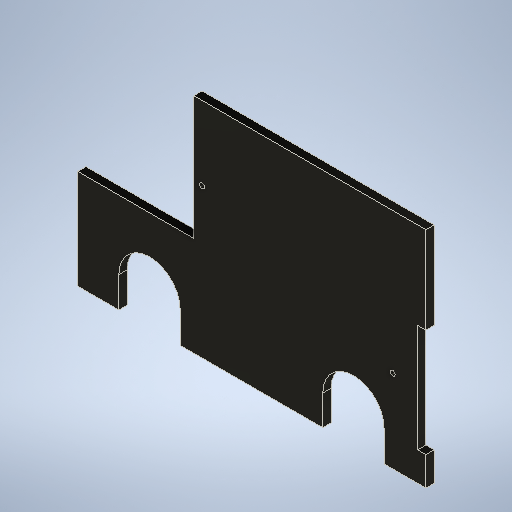
# Autodesk Inventor part: SIDE_1
Saved by Autodesk Inventor 2025.3 (Build 293356030, 356C)
## iProperties
Created: 2026-06-30
Part Number: SIDE_1
Material: ABS Plastic
Document SubType Name: Modeling
Designer: user
Density: 1.06 g/cm^3
Appearance: Gunmetal
Author: user
Autodesk Inventor part; units mm, degrees
ref_plane "YZ Plane" through (0, 0, 0) normal (1, 0, 0) x (0, 1, 0)
ref_plane "XZ Plane" through (0, 0, 0) normal (0, 1, 0) x (-1, 0, 0)
ref_plane "XY Plane" through (0, 0, 0) normal (0, 0, 1) x (1, 0, 0)
sketch "Sketch1" plane through (0, 0, 0) normal (0, 0, 1) x (1, 0, 0)
  line L0 (210, -0.4421) -> (210, 134.5579)
  line L1 (210, 134.5579) -> (70, 134.5579)
  line L2 (0, 60) -> (0, 0)
  line L3 (70, 60) -> (0, 60)
  line L4 (0, 60) -> (0, 0)
  line L5 (70, 60) -> (70, 134.5579)
  line L6 (0, 0) -> (24.7692, 0)
  line L7 (70, -0.4421) -> (70, 134.5579) construction
  arc A0 (184.7692, 18.0579) -> (147.7692, 18.0579) centre (166.2692, 18.0579) ccw
  line L8 (147.7692, 0) -> (147.7692, 18.0579)
  line L9 (184.7692, -0.4421) -> (184.7692, 18.0579)
  arc A1 (61.7692, 18.5) -> (24.7692, 18.5) centre (43.2692, 18.5) ccw
  line L10 (24.7692, 0) -> (24.7692, 18.5)
  line L11 (61.7692, 0) -> (61.7692, 18.5)
  line L12 (210, 17.0579) -> (205, 17.0579)
  line L13 (205, 17.0579) -> (205, 82.0579)
  line L14 (205, 82.0579) -> (210, 82.0579)
  line L15 (210, 82.0579) -> (210, 17.0579)
  line L16 (184.7692, -0.4421) -> (210, -0.4421)
  line L17 (61.7692, 0) -> (147.7692, 0)
  dimension "d14" = 210
  dimension "d15" = 70
  dimension "d17" = 37
  dimension "d19" = 37
  dimension "d23" = 5
  dimension "d24" = 65
  dimension "d28" = 52.5
  dimension "d48" = 135
  dimension "d51" = 18.5
  dimension "d52" = 18.5
  dimension "d54" = 18.5
  dimension "d55" = 60
  dimension "d60" = 18.5
  dimension "d61" = 123
  constraints: 36 end point, 6 parallel, 4 point on circle, 3 horizontal, 3 vertical, 2 centre point, 2 perpendicular, 1 point on line
  measures "d14" distance between parallel lines of L2 L0
  measures "d15" distance of L3.start L2.start
  measures "d17" distance between parallel lines of L9 L8
  measures "d19" distance between parallel lines of L11 L10
  measures "d23" distance of L13.end L14.end
  measures "d24" distance of L12.end L13.end
  measures "d28" distance between parallel lines of L14 L1
  measures "d48" distance of L0.start L0.end
  measures "d51" radius of A0
  measures "d52" radius of A1
  measures "d54" distance of L9.start L9.end
  measures "d55" distance of L2.start L2.end
  measures "d60" vertical distance of L2.end A1.centre
  measures "d61" horizontal distance of A1.centre A0.centre
extrude "Extrusion1" add sketch "Sketch1" along normal blind 5 contours L16 L9 A0 L8 L17 L11 A1 L10 L6 L2 L3 L5 L1 L0 L14 L13 L12
sketch "Sketch2" plane through (0, 0, 5) normal (0, 0, 1) x (1, 0, 0)
  line L0 (205, 17.0579) -> (205, 82.0579) projected
  line L1 (210, 17.0579) -> (205, 17.0579) projected
  point P0 (0, 0)
  point P1 (190, 49.5579)
  dimension "d36" = 15
  dimension "d37" = 32.5
  measures "d36" distance from line of L0 point (190, 49.558)
  measures "d37" distance from line of L1 point (190, 49.558)
hole "Hole1" at (190, 49.5579, 5) direction (0, 0, -1) diameter 3 end through all
sketch "Sketch3" plane through (0, 0, 5) normal (0, 0, 1) x (1, 0, 0)
  line L0 (70, 134.5579) -> (70, 60) projected
  line L1 (70, 60) -> (0, 60) projected
  point P0 (0, 0)
  point P1 (75, 90)
  dimension "d45" = 5
  dimension "d46" = 30
  measures "d45" distance from line of L0 point (75, 90)
  measures "d46" distance from line of point (75, 90) L1
hole "Hole2" at (75, 90, 5) direction (0, 0, -1) diameter 3 end through all
body "Solid1"
